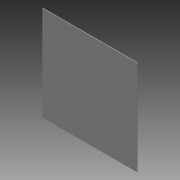
# Autodesk Inventor part: GE-13025-01
Saved by Autodesk Inventor 2013 (Build 170138000, 138)
## iProperties
Created: 2013-01-06
Part Number: GE-13025-01
Material: Steel
Document SubType Name: Modeling
Designer: Phillip
Density: 1 g/cm^3
Author: Phillip
Autodesk Inventor part; units mm, degrees
ref_plane "YZ Plane" through (0, 0, 0) normal (1, 0, 0) x (0, 1, 0)
ref_plane "XZ Plane" through (0, 0, 0) normal (0, 1, 0) x (-1, 0, 0)
ref_plane "XY Plane" through (0, 0, 0) normal (0, 0, 1) x (1, 0, 0)
sketch "Sketch1" plane through (0, 0, 0) normal (0, 0, 1) x (1, 0, 0)
  line L0 (0, 0) -> (609.6, 0)
  line L1 (609.6, 0) -> (609.6, 609.6)
  line L2 (609.6, 609.6) -> (0, 609.6)
  line L3 (0, 609.6) -> (0, 0)
  dimension "d0" = 609.6
  dimension "d1" = 609.6
  constraints: 8 end point, 2 parallel, 1 horizontal, 1 perpendicular
  measures "d0" distance of L2.end L1.end
  measures "d1" distance of L1.end L0.end
extrude "Extrusion1" add sketch "Sketch1" against normal blind 3.048
body "Solid1"
